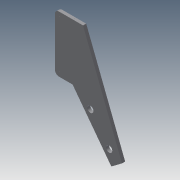
# Autodesk Inventor part: packa_sablona
Saved by Autodesk Inventor 2013 (Build 170138000, 138)
## iProperties
Created: 2013-02-02
Part Number: packa_sablona
Material: Generic
Document SubType Name: Modeling
Designer: idle-rug
Density: 1 g/cm^3
Author: idle-rug
Autodesk Inventor part; units mm, degrees
ref_plane "YZ Plane" through (0, 0, 0) normal (1, 0, 0) x (0, 1, 0)
ref_plane "XZ Plane" through (0, 0, 0) normal (0, 1, 0) x (-1, 0, 0)
ref_plane "XY Plane" through (0, 0, 0) normal (0, 0, 1) x (1, 0, 0)
sketch "Sketch2" plane through (0, 0, 0) normal (0, 1, 0) x (-1, 0, 0)
  line L0 (0.0014, 0.0009) -> (-14.9986, -19.9991)
  line L1 (0.0014, 0.0009) -> (-7.9986, 0.0009)
  line L2 (0.0014, 37.0009) -> (0.0014, 0.0009)
  line L3 (0.0014, 37.0009) -> (-7.9986, 0.0009)
  line L4 (-7.9986, 0.0009) -> (-20.8467, -17.1298)
  circle A0 centre (-8.4986, -5.9991) radius 1.5
  circle A1 centre (-17.4986, -17.9991) radius 1.5
  line L5 (-21.0986, -22.7991) -> (-18.5386, -24.7191)
  line L6 (-20.8467, -17.1298) -> (-23.6586, -20.8791)
  line L7 (-23.6586, -20.8791) -> (-18.5386, -24.7191)
  line L8 (-18.5386, -24.7191) -> (-14.9986, -19.9991)
  point P0 (0, 0)
  dimension "d4" = 3
  dimension "d5" = 3
  constraints: 18 end point, 2 centre point, 1 collinear, 1 horizontal, 1 parallel, 1 perpendicular
  measures "d4" diameter of A0
  measures "d5" diameter of A1
extrude "Extrusion1" add sketch "Sketch2" along normal blind 2
sketch "Sketch3" plane through (0, 2, 0) normal (0, 1, 0) x (1, 0, 0)
  line L0 (-0.0014, -0.0009) -> (-0.0014, -37.0009) projected
  line L1 (-0.0014, -37.0009) -> (7.9986, -0.0009) projected
  line L2 (7.9986, -0.0009) -> (23.6586, 20.8791) projected
  line L3 (-0.0014, -37.0009) -> (9.9986, -37.0009)
  line L4 (9.9986, -37.0009) -> (23.6586, 20.8791)
  point P0 (0, 0)
  dimension "d8" = 10
  constraints: 4 end point, 1 perpendicular
  measures "d8" distance of L0.end L3.end
extrude "Extrusion2" add sketch "Sketch3" against normal blind 2
sketch "Sketch4" plane through (0, 2, 0) normal (0, 1, 0) x (1, 0, 0)
  line L0 (-0.0014, -37.0009) -> (9.9986, -37.0009) projected
  line L1 (9.9986, -37.0009) -> (23.6586, 20.8791) projected
  line L2 (4.9986, -37.0009) -> (23.6586, 20.8791)
  line L3 (4.9986, -37.0009) -> (9.9986, -37.0009)
  line L4 (9.9986, -37.0009) -> (23.6586, 20.8791)
  point P0 (0, 0)
  dimension "d13" = 5
  constraints: 6 end point, 2 collinear, 1 midpoint
  measures "d13" distance of L0.start L2.start
extrude "Extrusion3" cut sketch "Sketch4" against normal blind 2
sketch "Sketch6" plane through (0, 0, 0) normal (0, -1, 0) x (1, 0, 0)
  line L0 (4.9986, 37.0009) -> (-0.0014, 37.0009) projected
  line L1 (-0.0014, 0.0009) -> (-0.0014, 37.0009) projected
  line L2 (-0.0014, 37.0009) -> (1.9986, 37.0009)
  line L3 (1.9986, 37.0009) -> (1.9986, 0)
  line L4 (1.9986, 0) -> (0, 0)
  line L5 (0, 0) -> (-0.0014, 37.0009)
  dimension "d16" = 2
  constraints: 8 end point, 1 parallel, 1 perpendicular, 1 point on line
  measures "d16" distance of L0.end L2.end
extrude "Extrusion4" add sketch "Sketch6" along normal blind 6
sketch "Sketch9" plane through (0, 0, 0) normal (0, -1, 0) x (1, 0, 0)
  circle A0 centre (17.4986, -17.9991) radius 1.5 projected
  circle A1 centre (8.4986, -5.9991) radius 1.5 projected
  line L0 (1.9986, 37.0009) -> (1.9986, 0) projected
  line L1 (1.9986, 0) -> (0, 0) projected
  line L2 (0, 0) -> (-0.0014, 37.0009) projected
  line L3 (-0.0014, 0.0009) -> (-0.0014, 37.0009) projected
  line L4 (18.5386, -24.7191) -> (-0.0014, 0.0009) projected
  line L5 (23.6586, -20.8791) -> (18.5386, -24.7191) projected
  line L6 (23.6586, -20.8791) -> (4.9986, 37.0009) projected
  line L7 (4.9986, 37.0009) -> (1.9986, 37.0009) projected
extrude "Extrusion5" cut sketch "Sketch9" against normal blind 0.5
sketch "Sketch11" plane through (0, 2, 0) normal (0, 1, 0) x (1, 0, 0)
  line L0 (4.9986, -37.0009) -> (23.6586, 20.8791) projected
  line L1 (-0.0014, -0.0009) -> (-0.0014, -37.0009) projected
  line L2 (-0.0014, -37.0009) -> (4.9986, -37.0009) projected
  line L3 (-0.0014, -37.0009) -> (-0.0014, -27.0009)
  line L4 (-0.0014, -27.0009) -> (4.9986, -27.0009)
  line L5 (4.9986, -27.0009) -> (23.6586, 20.8791)
  line L6 (23.6586, 20.8791) -> (4.9986, -37.0009)
  line L7 (4.9986, -37.0009) -> (-0.0014, -37.0009)
  point P0 (0, 0)
  dimension "d21" = 10
  dimension "d22" = 5
  constraints: 10 end point, 2 collinear, 1 perpendicular, 1 point on line
  measures "d21" distance of L1.end L3.end
  measures "d22" distance of L3.end L4.end
extrude "Extrusion6" cut sketch "Sketch11" against normal blind 1.5
sketch "Sketch12" plane through (0, 0.5, 0) normal (0, 1, 0) x (1, 0, 0)
  line L0 (-0.0014, -37.0009) -> (-0.001, -27.0009) projected
  line L1 (1.9986, -37.0009) -> (-0.0014, -37.0009) projected
  line L2 (1.9986, -27.0009) -> (1.9986, -37.0009) projected
  line L3 (-0.001, -27.0009) -> (1.9986, -27.0009) projected
  point P0 (0, 0)
extrude "Extrusion7" cut sketch "Sketch12" against normal blind 1.5
sketch "Sketch13" plane through (0, -1, 0) normal (0, 1, 0) x (1, 0, 0)
  line L0 (-0.0014, -37.0009) -> (-0.001, -27.0009) projected
  line L1 (1.9986, -37.0009) -> (-0.0014, -37.0009) projected
  line L2 (1.9986, -27.0009) -> (1.9986, -37.0009) projected
  line L3 (-0.001, -27.0009) -> (1.9986, -27.0009) projected
  point P0 (0, 0)
extrude "Extrusion8" cut sketch "Sketch13" against normal blind 10
fillet "Fillet1" radius 2 1 edges at (0.9988, -6, 27.0009)
fillet "Fillet2" radius 2 1 edges at (0.9993, -6, 0)
sketch "Sketch15" plane through (1.9986, 0.5, 27.0009) normal (1, 0, 0) x (0, 0, -1)
  arc A0 (25.0009, -6.5) -> (27.0009, -4.5) centre (25.0009, -4.5) ccw projected
  line L0 (27.0009, -4.5) -> (27.0009, 0) projected
  line L1 (27.0009, 0) -> (0, 0) projected
  line L2 (0, 0) -> (0, -4.5) projected
  arc A1 (0, -4.5) -> (2, -6.5) centre (2, -4.5) ccw projected
  line L3 (25.0009, -6.5) -> (2, -6.5) projected
  point P0 (27.0009, -0.5)
extrude "Extrusion9" cut sketch "Sketch15" against normal blind 10
sketch "Sketch16" plane through (-0.0014, 0.5, 0.0009) normal (-1, 0, 0) x (0, 0, 1)
  line L0 (27, 0) -> (27, 1.5) projected
  line L1 (0, 1.5) -> (27, 1.5) projected
  line L2 (0, 0) -> (0, 1.5) projected
  line L3 (0, 0) -> (27, 0) projected
  point P0 (-0.0009, -0.5)
extrude "Extrusion10" add sketch "Sketch16" along normal blind 6.5
sketch "Sketch17" plane through (0, 0.5, 0) normal (0, -1, 0) x (1, 0, 0)
  line L0 (-0.0014, 0.0009) -> (-6.5014, 0.0009) projected
  line L1 (-6.5014, 0.0009) -> (-0.0014, 0.0009)
  line L2 (-0.0014, 0.0009) -> (-0.0014, 26.9909)
  line L3 (-0.0014, 27.0009) -> (-0.0114, 27.0009)
  line L4 (-0.0014, 0.0009) -> (-0.0114, 0.0009)
  line L5 (-0.0114, 0.0009) -> (-0.0114, 27.0009)
  line L6 (-0.0014, 27.0009) -> (-0.0014, 26.9909)
  line L7 (-0.0014, 27.0009) -> (-0.0014, 0.0009)
  line L8 (-0.0014, 0.0009) -> (-0.0114, 0.0009)
  line L9 (-0.0114, 0.0009) -> (-0.0114, 27.0009)
  dimension "d43" = 0.01
  constraints: 18 end point, 3 collinear, 1 parallel, 1 point on line
  measures "d43" distance of L0.start L4.end
sketch "Sketch19" plane through (-6.5014, 0.5, 0.0009) normal (-1, 0, 0) x (0, 0, 1)
  line L0 (27, 0) -> (27, 1.5) projected
  line L1 (27, 1.5) -> (0, 1.5) projected
  line L2 (0, 1.5) -> (0, 0) projected
  line L3 (0, 0) -> (27, 0) projected
  point P0 (-0.0009, -0.5)
extrude "Extrusion11" add sketch "Sketch19" along normal blind 2
fillet "Fillet3" radius 2 1 edges at (-8.5014, 1.25, 27.0009)
fillet "Fillet4" radius 2 1 edges at (-8.5014, 1.25, 0.0009)
extrude "Extrusion12" cut sketch "Sketch17" against normal blind 10
sketch "Sketch20" plane through (0, 0.5, 0) normal (0, -1, 0) x (1, 0, 0)
  arc A0 (-6.5014, 27.0009) -> (-8.5014, 25.0009) centre (-6.5014, 25.0009) ccw projected
  arc A1 (-8.5014, 2.0009) -> (-6.5014, 0.0009) centre (-6.5014, 2.0009) ccw projected
  circle A2 centre (-6.5014, 25.0009) radius 0.1
  circle A3 centre (-6.5014, 2.0009) radius 0.1
  point P0 (0, 0)
  dimension "d46" = 0.2
  dimension "d47" = 0.2
  constraints: 2 centre point, 2 coincident
  measures "d46" diameter of A2
  measures "d47" diameter of A3
extrude "Extrusion13" cut sketch "Sketch20" against normal blind 10
body "Solid1"
